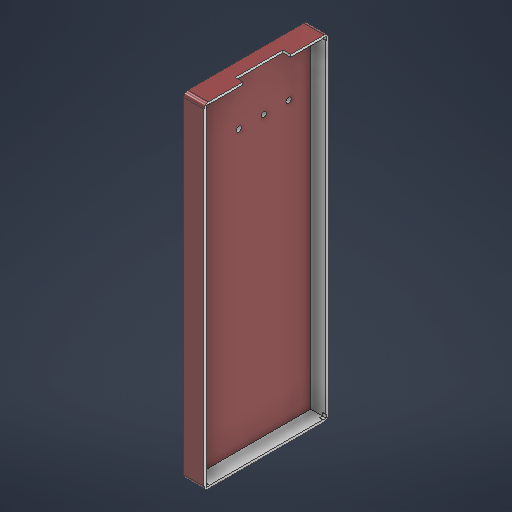
# Autodesk Inventor part: cDAQ_Lid_Box
Saved by Autodesk Inventor 2027 (Build 310192000, 192)
## iProperties
Created: 2026-05-08
Part Number: cDAQ_Lid_Box
Material: Generic
Document SubType Name: Modeling
Designer: giese
Density: 1 g/cm^3
Appearance: Default
Author: giese
Autodesk Inventor part; units mm, degrees
ref_plane "YZ Plane" through (0, 0, 0) normal (1, 0, 0) x (0, 1, 0)
ref_plane "XZ Plane" through (0, 0, 0) normal (0, 1, 0) x (-1, 0, 0)
ref_plane "XY Plane" through (0, 0, 0) normal (0, 0, 1) x (1, 0, 0)
sketch "Sketch1" plane through (0, 0, 0) normal (1, 0, 0) x (0, 1, 0)
  line L0 (50.7569, 48.4212) -> (-198.7981, 48.4212)
  line L1 (-198.7981, 48.4212) -> (-198.7981, -44.2888)
  line L2 (-198.7981, -44.2888) -> (50.7569, -44.2888)
  line L3 (50.7569, -44.2888) -> (50.7569, 48.4212)
  point P0 (0, 0)
  dimension "d0" = 92.71
  dimension "d1" = 249.555
  constraints: 8 end point, 2 parallel, 1 horizontal, 1 perpendicular
  measures "d0" distance of L2.end L0.start
  measures "d1" distance of L0.start L0.end
extrude "Extrusion1" add sketch "Sketch1" along normal blind 15.24
sketch "Sketch2" plane through (15.24, 0, 0) normal (1, 0, 0) x (0, 0, -1)
  line L0 (-46.5162, 48.8519) -> (42.3838, 48.8519)
  line L1 (42.3838, 48.8519) -> (42.3838, -196.8931)
  line L2 (42.3838, -196.8931) -> (-46.5162, -196.8931)
  line L3 (-46.5162, -196.8931) -> (-46.5162, 48.8519)
  line L4 (-48.4212, 50.7569) -> (-48.4212, -198.7981) projected
  line L5 (-48.4212, -198.7981) -> (44.2888, -198.7981) projected
  point P0 (0, 0)
  dimension "d4" = 88.9
  dimension "d5" = 245.745
  dimension "d6" = 1.905
  dimension "d7" = 1.905
  constraints: 8 end point, 2 parallel, 1 horizontal, 1 perpendicular
  measures "d4" distance of L0.start L0.end
  measures "d5" distance of L0.end L1.end
  measures "d6" distance between parallel lines of L4 L3
  measures "d7" distance between parallel lines of L5 L2
extrude "Extrusion2" cut sketch "Sketch2" against normal blind 11.43
sketch "Sketch3" plane through (0, 0, 0) normal (-1, 0, 0) x (0, 0, 1)
  circle A0 centre (-26.0008, 10.5233) radius 2
  line L0 (-44.2888, -198.7981) -> (-44.2888, 50.7569) projected
  line L1 (-44.2888, 50.7569) -> (48.4212, 50.7569) projected
  circle A1 centre (-7.502, 10.5233) radius 2
  circle A2 centre (10.9969, 10.5233) radius 2
  point P0 (0, 0)
  dimension "d10" = 18.288
  dimension "d11" = 40.2336
  dimension "d12" = 40.2336
  dimension "d13" = 18.4988
  dimension "d14" = 4
  dimension "d15" = 4
  dimension "d16" = 40.2336
  dimension "d17" = 18.4988
  dimension "d18" = 36.9976
  dimension "d21" = 4
  constraints: 3 centre point
  measures "d10" distance from line of L0 A0.centre
  measures "d11" distance from line of L1 A0.centre
  measures "d12" distance from line of L1 A1.centre
  measures "d13" distance of A0.centre A1.centre
  measures "d14" diameter of A1
  measures "d15" diameter of A2
  measures "d16" distance from line of L1 A2.centre
  measures "d17" distance of A1.centre A2.centre
  measures "d18" distance of A0.centre A2.centre
  measures "d21" diameter of A0
extrude "Extrusion3" cut sketch "Sketch3" against normal blind 3.81
sketch "Sketch6" plane through (0, 50.7569, 48.4212) normal (0, 1, 0) x (1, 0, 0)
  line L0 (15.24, 1.905) -> (15.24, 90.805) projected
  line L1 (9.4234, 28.9459) -> (15.24, 28.9459)
  line L2 (15.24, 28.9459) -> (15.24, 64.516)
  line L3 (15.24, 64.516) -> (9.4234, 64.516)
  line L4 (9.4234, 64.516) -> (9.4234, 28.9459)
  line L5 (0, 92.71) -> (15.24, 92.71) projected
  point P0 (0, 48.4212)
  point P1 (12.3317, 64.516)
  point P2 (12.3317, 28.9459)
  dimension "d30" = 5.8166
  dimension "d31" = 35.5701
  dimension "d32" = 28.194
  constraints: 8 end point, 2 midpoint, 2 parallel, 1 horizontal, 1 perpendicular, 1 point on line
  measures "d30" distance between parallel lines of L0 L4
  measures "d31" distance of point (12.332, 64.516) point (12.332, 28.946)
  measures "d32" distance between parallel lines of L5 L3
extrude "Extrusion5" cut sketch "Sketch6" against normal blind 3.81
fillet "Fillet1" radius 3.175 4 edges at (7.62, 50.7569, -44.2888) (7.62, 50.7569, 48.4212) (7.62, -198.7981, 48.4212) (7.62, -198.7981, -44.2888)
sketch "Sketch7" plane through (15.24, 0, 0) normal (1, 0, 0) x (0, 0, -1)
  line L0 (-46.5162, -196.8931) -> (-46.5162, 48.8519) projected
  line L1 (-46.5162, 46.5659) -> (-46.5162, 48.8519)
  line L2 (-46.5162, 48.8519) -> (-44.2302, 48.8519)
  line L3 (-44.2302, 48.8519) -> (-44.2302, 49.1059)
  line L4 (-44.2302, 49.1059) -> (-46.7702, 49.1059)
  line L5 (-46.7702, 49.1059) -> (-46.7702, 46.5659)
  line L6 (-46.7702, 46.5659) -> (-46.5162, 46.5659)
  line L7 (-46.5162, -194.6071) -> (-46.5162, -196.8931)
  line L8 (42.3838, -196.8931) -> (-46.5162, -196.8931) projected
  line L9 (-44.2302, -196.8931) -> (-44.2302, -197.1471)
  line L10 (-44.2302, -197.1471) -> (-46.7702, -197.1471)
  line L11 (-46.7702, -197.1471) -> (-46.7702, -194.6071)
  line L12 (-46.7702, -194.6071) -> (-46.5162, -194.6071)
  line L13 (42.3838, 48.8519) -> (42.3838, -196.8931) projected
  line L14 (42.3838, -194.6071) -> (42.3838, -196.8931)
  line L15 (42.3838, -196.8931) -> (40.0978, -196.8931)
  line L16 (40.0978, -197.1471) -> (40.0978, -196.8931)
  line L17 (42.3838, -196.8931) -> (42.3838, -194.6071)
  line L18 (42.3838, -194.6071) -> (42.6378, -194.6071)
  line L19 (42.6378, -194.6071) -> (42.6378, -197.1471)
  line L20 (42.6378, -197.1471) -> (40.0978, -197.1471)
  line L21 (-46.5162, 48.8519) -> (42.3838, 48.8519) projected
  line L22 (40.0978, 48.8519) -> (42.3838, 48.8519)
  line L23 (42.3838, 48.8519) -> (42.3838, 46.5659)
  line L24 (42.3838, 46.5659) -> (42.6378, 46.5659)
  line L25 (42.6378, 46.5659) -> (42.6378, 49.1059)
  line L26 (42.6378, 49.1059) -> (40.0978, 49.1059)
  line L27 (40.0978, 49.1059) -> (40.0978, 48.8519)
  point P0 (0, 0)
  point P1 (-44.2302, 48.9789)
  dimension "d34" = 0.254
  dimension "d35" = 0.254
  dimension "d36" = 2.54
  dimension "d37" = 2.54
  dimension "d38" = 0.254
  dimension "d39" = 0.254
  dimension "d40" = 2.54
  dimension "d41" = 2.54
  dimension "d42" = 0.254
  dimension "d43" = 0.254
  dimension "d44" = 2.54
  dimension "d45" = 2.54
  dimension "d46" = 0.254
  dimension "d47" = 0.254
  dimension "d48" = 2.54
  dimension "d49" = 2.54
  constraints: 48 end point, 14 perpendicular, 7 point on line, 3 collinear, 3 vertical, 2 horizontal, 1 midpoint
  measures "d34" distance between parallel lines of L4 L2
  measures "d35" distance between parallel lines of L0 L5
  measures "d36" distance between parallel lines of L4 L6
  measures "d37" distance from line of point (-44.23, 48.979) L5
  measures "d38" distance between parallel lines of L11 L0
  measures "d39" distance between parallel lines of L8 L10
  measures "d40" distance between parallel lines of L11 L9
  measures "d41" distance between parallel lines of L10 L12
  measures "d42" distance between parallel lines of L8 L20
  measures "d43" distance between parallel lines of L13 L19
  measures "d44" distance between parallel lines of L20 L18
  measures "d45" distance between parallel lines of L16 L19
  measures "d46" distance between parallel lines of L21 L26
  measures "d47" distance between parallel lines of L13 L25
  measures "d48" distance between parallel lines of L26 L24
  measures "d49" distance between parallel lines of L27 L25
extrude "Extrusion6" cut sketch "Sketch7" against normal blind 2.54 contours L8 L9 L10 L11 L12 L0 | L6 L5 L4 L3 L2 L0 | L8 L13 L18 L19 L20 L16 | L27 L26 L25 L24 L13 L21
body "Solid1"
